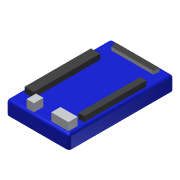
# Autodesk Inventor part: Digital Sidecar
Saved by Autodesk Inventor 2013 (Build 170138000, 138)
## iProperties
Created: 2013-12-22
Part Number: Digital Sidecar
Material: Generic
Document SubType Name: Modeling
Designer: Nemo
Mass: 113.398 g
Surface Area: 344.174 cm^2
Volume: 173.536 cm^3
Density: 0.653456 g/cm^3
Author: Nemo
Autodesk Inventor part; units mm, degrees
ref_plane "YZ Plane" through (0, 0, 0) normal (1, 0, 0) x (0, 1, 0)
ref_plane "XZ Plane" through (0, 0, 0) normal (0, 1, 0) x (-1, 0, 0)
ref_plane "XY Plane" through (0, 0, 0) normal (0, 0, 1) x (1, 0, 0)
sketch "DB37" plane through (0, 0, 0) normal (0, 0, 1) x (1, 0, 0)
  circle A0 centre (16.6221, 54.9047) radius 0.4445
  circle A1 centre (8.3121, 54.9047) radius 0.4445
  circle A2 centre (9.6971, 52.0647) radius 0.4445
  circle A3 centre (11.0821, 54.9047) radius 0.4445
  circle A4 centre (12.4671, 52.0647) radius 0.4445
  circle A5 centre (15.2371, 52.0647) radius 0.4445
  circle A6 centre (18.0071, 52.0647) radius 0.4445
  circle A7 centre (13.8521, 54.9047) radius 0.4445
  circle A8 centre (-4.1529, 52.0647) radius 0.4445
  circle A9 centre (-2.7679, 54.9047) radius 0.4445
  circle A10 centre (-1.3829, 52.0647) radius 0.4445
  circle A11 centre (0.0021, 54.9047) radius 0.4445
  circle A12 centre (1.3871, 52.0647) radius 0.4445
  circle A13 centre (2.7721, 54.9047) radius 0.4445
  circle A14 centre (5.5421, 54.9047) radius 0.4445
  circle A15 centre (4.1571, 52.0647) radius 0.4445
  circle A16 centre (6.9271, 52.0647) radius 0.4445
  circle A17 centre (-18.0029, 52.0647) radius 0.4445
  circle A18 centre (-19.3879, 54.9047) radius 0.4445
  circle A19 centre (-20.7729, 52.0647) radius 0.4445
  arc A20 (-25.7175, 50.671) -> (-24.9592, 50.0347) centre (-24.9592, 50.8047) ccw
  line L0 (26.6669, 56.031) -> (25.7218, 50.671)
  arc A21 (26.6669, 56.031) -> (25.9086, 56.9347) centre (25.9086, 56.1647) ccw
  arc A22 (24.9635, 50.0347) -> (25.7218, 50.671) centre (24.9635, 50.8047) ccw
  circle A23 centre (22.1621, 54.9047) radius 0.4445
  circle A24 centre (24.9321, 54.9047) radius 0.4445
  circle A25 centre (23.5471, 52.0647) radius 0.4445
  circle A26 centre (19.3921, 54.9047) radius 0.4445
  circle A27 centre (20.7771, 52.0647) radius 0.4445
  line L1 (24.9635, 50.0347) -> (-24.9592, 50.0347)
  line L2 (-25.9043, 56.9347) -> (25.9086, 56.9347)
  circle A28 centre (-5.5379, 54.9047) radius 0.4445
  circle A29 centre (-6.9229, 52.0647) radius 0.4445
  circle A30 centre (-8.3079, 54.9047) radius 0.4445
  circle A31 centre (-9.6929, 52.0647) radius 0.4445
  circle A32 centre (-11.0779, 54.9047) radius 0.4445
  circle A33 centre (-12.4629, 52.0647) radius 0.4445
  circle A34 centre (-13.8479, 54.9047) radius 0.4445
  circle A35 centre (-15.2329, 52.0647) radius 0.4445
  circle A36 centre (-16.6179, 54.9047) radius 0.4445
  circle A37 centre (-24.9279, 54.9047) radius 0.4445
  circle A38 centre (-23.5429, 52.0647) radius 0.4445
  line L3 (-25.7175, 50.671) -> (-26.6626, 56.031)
  arc A39 (-25.9043, 56.9347) -> (-26.6626, 56.031) centre (-25.9043, 56.1647) ccw
  circle A40 centre (-22.1579, 54.9047) radius 0.4445
  point P0 (0.0021, 53.4969)
sketch "Sketch2" plane through (0, 0, 0) normal (0, 1, 0) x (-1, 0, 0)
  line L0 (-38.1, 63.5) -> (38.1, 63.5)
  line L1 (38.1, 63.5) -> (38.1, -63.5)
  line L2 (38.1, -63.5) -> (-38.1, -63.5)
  line L3 (-38.1, -63.5) -> (-38.1, 63.5)
  point P0 (0, 0)
  point P1 (0, 63.5)
  point P2 (-38.1, 0)
  dimension "d0" = 76.2
  dimension "d2" = 127
  constraints: 8 end point, 2 midpoint, 2 parallel, 1 horizontal, 1 horizontal alignment, 1 perpendicular, 1 vertical alignment
  measures "d0" distance of L0.start L0.end
  measures "d2" distance of L2.end L0.start
extrude "Extrusion1" add sketch "Sketch2" along normal blind 16.51
sketch "Sketch3" plane through (0, 16.51, 0) normal (0, 1, 0) x (1, 0, 0)
  circle A0 centre (16.62, 55.8173) radius 0.4445
  circle A1 centre (8.31, 55.8173) radius 0.4445
  circle A2 centre (9.695, 52.9773) radius 0.4445
  circle A3 centre (11.08, 55.8173) radius 0.4445
  circle A4 centre (12.465, 52.9773) radius 0.4445
  circle A5 centre (15.235, 52.9773) radius 0.4445
  circle A6 centre (18.005, 52.9773) radius 0.4445
  circle A7 centre (13.85, 55.8173) radius 0.4445
  circle A8 centre (-4.155, 52.9773) radius 0.4445
  circle A9 centre (-2.77, 55.8173) radius 0.4445
  circle A10 centre (-1.385, 52.9773) radius 0.4445
  circle A11 centre (0, 55.8173) radius 0.4445
  circle A12 centre (1.385, 52.9773) radius 0.4445
  circle A13 centre (2.77, 55.8173) radius 0.4445
  circle A14 centre (5.54, 55.8173) radius 0.4445
  circle A15 centre (4.155, 52.9773) radius 0.4445
  circle A16 centre (6.925, 52.9773) radius 0.4445
  circle A17 centre (-18.005, 52.9773) radius 0.4445
  circle A18 centre (-19.39, 55.8173) radius 0.4445
  circle A19 centre (-20.775, 52.9773) radius 0.4445
  arc A20 (-25.7197, 51.5836) -> (-24.9614, 50.9473) centre (-24.9614, 51.7173) ccw
  line L0 (26.6648, 56.9436) -> (25.7197, 51.5836)
  arc A21 (26.6648, 56.9436) -> (25.9065, 57.8473) centre (25.9065, 57.0773) ccw
  arc A22 (24.9614, 50.9473) -> (25.7197, 51.5836) centre (24.9614, 51.7173) ccw
  circle A23 centre (22.16, 55.8173) radius 0.4445
  circle A24 centre (24.93, 55.8173) radius 0.4445
  circle A25 centre (23.545, 52.9773) radius 0.4445
  circle A26 centre (19.39, 55.8173) radius 0.4445
  circle A27 centre (20.775, 52.9773) radius 0.4445
  line L1 (24.9614, 50.9473) -> (-24.9614, 50.9473)
  line L2 (-25.9065, 57.8473) -> (25.9065, 57.8473)
  circle A28 centre (-5.54, 55.8173) radius 0.4445
  circle A29 centre (-6.925, 52.9773) radius 0.4445
  circle A30 centre (-8.31, 55.8173) radius 0.4445
  circle A31 centre (-9.695, 52.9773) radius 0.4445
  circle A32 centre (-11.08, 55.8173) radius 0.4445
  circle A33 centre (-12.465, 52.9773) radius 0.4445
  circle A34 centre (-13.85, 55.8173) radius 0.4445
  circle A35 centre (-15.235, 52.9773) radius 0.4445
  circle A36 centre (-16.62, 55.8173) radius 0.4445
  circle A37 centre (-24.93, 55.8173) radius 0.4445
  circle A38 centre (-23.545, 52.9773) radius 0.4445
  line L3 (-25.7197, 51.5836) -> (-26.6648, 56.9436)
  arc A39 (-25.9065, 57.8473) -> (-26.6648, 56.9436) centre (-25.9065, 57.0773) ccw
  circle A40 centre (-22.16, 55.8173) radius 0.4445
  point P0 (0, 0)
  constraints: 1 other
extrude "Extrusion2" add sketch "Sketch3" along normal blind 4.064 separate body
sketch "Sketch4" plane through (0, 16.51, 0) normal (0, 1, 0) x (1, 0, 0)
  line L0 (-33.2386, 34.4509) -> (-22.0901, 34.4509)
  line L1 (-22.0901, 34.4509) -> (-22.0901, -46.0879)
  line L2 (-22.0901, -46.0879) -> (-33.2386, -46.0879)
  line L3 (-33.2386, -46.0879) -> (-33.2386, 34.4509)
  line L4 (26.7329, 34.4509) -> (34.0372, 34.4509)
  line L5 (34.0372, 34.4509) -> (34.0372, -40.9792)
  line L6 (34.0372, -40.9792) -> (26.7329, -40.9792)
  line L7 (26.7329, -40.9792) -> (26.7329, 34.4509)
  point P0 (0, 0)
  constraints: 16 end point, 4 parallel, 2 horizontal, 2 perpendicular
extrude "Extrusion3" add sketch "Sketch4" along normal blind 6.35 separate body
sketch "Sketch5" plane through (0, 16.51, 0) normal (0, 1, 0) x (1, 0, 0)
  line L0 (12.9181, -48.6758) -> (33.6935, -48.6758)
  line L1 (33.6935, -48.6758) -> (33.6935, -59.8626)
  line L2 (33.6935, -59.8626) -> (12.9181, -59.8626)
  line L3 (12.9181, -59.8626) -> (12.9181, -48.6758)
  line L4 (-15.9811, -49.4749) -> (-7.0583, -49.4749)
  line L5 (-7.0583, -49.4749) -> (-7.0583, -60.928)
  line L6 (-7.0583, -60.928) -> (-15.9811, -60.928)
  line L7 (-15.9811, -60.928) -> (-15.9811, -49.4749)
  point P0 (0, 0)
  constraints: 16 end point, 4 parallel, 2 horizontal, 2 perpendicular
extrude "Extrusion4" add sketch "Sketch5" along normal blind 9.525 separate body
fillet "Fillet1" radius 3.175 8 edges at (-38.1, 8.255, 63.5) (38.1, 8.255, 63.5) (38.1, 8.255, -63.5) (-38.1, 8.255, -63.5) (-38.1, 16.51, 0) (0, 16.51, -63.5) (38.1, 16.51, 0) (0, 16.51, 63.5)
body "Solid1"
body "Solid2"
body "Solid3"
body "Solid4"
